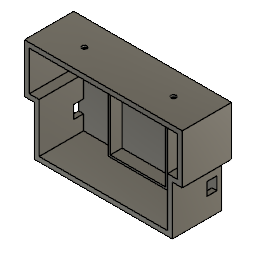
cajon v4 (Autodesk Fusion 360 design; units mm, degrees)
Autodesk Fusion 360 part; units mm, degrees
sketch "Boceto1" plane through (0, 0, 0) normal (0, 1, 0) x (1, 0, 0)
  line L0 (-60, 40) -> (80, 40)
  line L1 (80, 40) -> (80, -10)
  line L2 (80, -10) -> (90, -10)
  line L3 (90, -10) -> (90, -60)
  line L4 (90, -60) -> (-70, -60)
  line L5 (-70, -60) -> (-70, -10)
  line L6 (-70, -10) -> (-60, -10)
  line L7 (-60, -10) -> (-60, 40)
  constraint horizontal L0
  constraint perpendicular L0 L1
  constraint perpendicular L1 L2
  constraint perpendicular L2 L3
  constraint perpendicular L3 L4
  constraint perpendicular L4 L5
  constraint perpendicular L5 L6
  constraint perpendicular L0 L7
extrude "Extruir1" add sketch "Boceto1" along normal blind 50
shell "Vaciado1" thickness 5 removed faces 1 at (-13.3333, 0, 43.3333)
sketch "Boceto2" plane through (0, 0, 0) normal (0, 1, 0) x (1, 0, 0)
  line L0 (75, 20) -> (80, 20)
  line L1 (80, 20) -> (80, 7)
  line L2 (80, 7) -> (75, 7)
  line L3 (75, 7) -> (75, 20)
  dimension "d4" = 13
  constraint horizontal L0
  constraint perpendicular L0 L1
  constraint perpendicular L1 L2
  constraint perpendicular L0 L3
  measures "d4" distance of L0.end L1.end
extrude "Extruir2" cut sketch "Boceto2" along normal blind 45
sketch "Boceto3" plane through (0, 0, 0) normal (0, 1, 0) x (1, 0, 0)
  line L0 (75, 20) -> (80, 20)
  line L1 (80, 20) -> (80, 7)
  line L2 (80, 7) -> (75, 7)
  line L3 (75, 7) -> (75, 20)
  dimension "d7" = 13
  constraint horizontal L0
  constraint perpendicular L0 L1
  constraint perpendicular L1 L2
  constraint perpendicular L0 L3
  measures "d7" distance of L0.end L1.end
extrude "Extruir3" add sketch "Boceto3" along normal blind 35
sketch "Boceto4" plane through (0, 0, 0) normal (0, 1, 0) x (1, 0, 0)
  line L0 (-60, 20) -> (-55, 20)
  line L1 (-55, 20) -> (-55, 7)
  line L2 (-55, 7) -> (-60, 7)
  line L3 (-60, 20) -> (-60, 7)
  dimension "d10" = 13
  constraint horizontal L0
  constraint perpendicular L0 L1
  constraint perpendicular L1 L2
  constraint perpendicular L2 L3
  measures "d10" distance of L0.end L1.end
extrude "Extruir4" cut sketch "Boceto4" along normal blind 45
sketch "Boceto5" plane through (0, 0, 0) normal (0, 1, 0) x (1, 0, 0)
  line L0 (-55, 20) -> (-55, 7)
  line L1 (-55, 7) -> (-60, 7)
  line L2 (-60, 7) -> (-60, 20)
  line L3 (-60, 20) -> (-55, 20)
  dimension "d13" = 13
  constraint vertical L0
  constraint perpendicular L0 L1
  constraint perpendicular L1 L2
  constraint perpendicular L0 L3
  measures "d13" distance of L0.start L0.end
extrude "Extruir5" add sketch "Boceto5" along normal blind 35
sketch "Boceto6" plane through (0, 0, 0) normal (0, 1, 0) x (1, 0, 0)
  line L0 (-19.9878, 34.6702, 35) -> (40.0122, 34.6702, 35)
  line L1 (40.0122, 34.6702, 35) -> (40.0122, -40.3298, 35)
  line L2 (40.0122, -40.3298, 35) -> (-19.9878, -40.3298, 35)
  line L3 (-19.9878, -40.3298, 35) -> (-19.9878, 34.6702, 35)
  dimension "d16" = 60
  dimension "d17" = 75
extrude "Extruir6" add sketch "Boceto6" along normal blind 10 contours L0 L1 L2 L3 in plane through (0, 35, 0) normal (0, 1, 0)
shell "Vaciado2" thickness 2 removed faces 1 at (0.0122, 35, -9.6702)
hole "Agujero1" at (-32.8621, 23.8094, 60) direction (0, 0, -1) diameter 5 depth 10 tip angle 118
hole "Agujero2" at (55.5835, 25.5103, 60) direction (0, 0, -1) diameter 5 depth 10 tip angle 118
